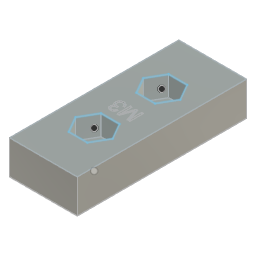
Joints v5 (Autodesk Fusion 360 design; units mm, degrees)
Autodesk Fusion 360 part; units mm, degrees
box "BoxPrimitive3" add length 5 width 10 height 25 placed x (0, 0, 1) y (1, 0, 0) z (0, 1, 0) at (0, 0, 0)
sketch "Sketch5" plane through (0, 0, 5) normal (0, 0, 1) x (-1, 0, 0)
  line L0 (0, -25) -> (0, 0)
  line L1 (0, 0) -> (-10, 0)
  line L2 (-10, 0) -> (-10, -25)
  line L3 (-10, -25) -> (0, -25)
  line L4 (-7.75, -7.5) -> (-6.375, -9.8816)
  line L5 (-6.375, -9.8816) -> (-3.625, -9.8816)
  line L6 (-3.625, -9.8816) -> (-2.25, -7.5)
  line L7 (-2.25, -7.5) -> (-3.625, -5.1184)
  line L8 (-3.625, -5.1184) -> (-6.375, -5.1184)
  line L9 (-6.375, -5.1184) -> (-7.75, -7.5)
  line L10 (-7.75, -17.5) -> (-6.375, -19.8816)
  line L11 (-6.375, -19.8816) -> (-3.625, -19.8816)
  line L12 (-3.625, -19.8816) -> (-2.25, -17.5)
  line L13 (-2.25, -17.5) -> (-3.625, -15.1184)
  line L14 (-3.625, -15.1184) -> (-6.375, -15.1184)
  line L15 (-6.375, -15.1184) -> (-7.75, -17.5)
  point P0 (-5, -17.5)
  point P1 (-5, -7.5)
  point P2 (-5, -17.5)
  point P3 (-5, -7.5)
  point P4 (-5, -17.5)
  point P5 (-5, -7.5)
  dimension "d23" = 2.75
  dimension "d24" = 2.75
  constraint coincident P4 P2
  constraint coincident P5 P3
  measures "d23" distance of L4.start P5
  measures "d24" distance of L10.start P4
extrude "Extrude3" cut sketch "Sketch5" against normal blind 3 contours L4 L5 L6 L7 L8 L9 | L10 L11 L12 L13 L14 L15
sketch "Sketch7" plane through (0, 0, 5) normal (0, 0, 1) x (-1, 0, 0)
  line L0 (-6.375, -19.8816) -> (-7.75, -17.5)
  line L1 (-7.75, -17.5) -> (-6.375, -15.1184)
  line L2 (-6.375, -15.1184) -> (-3.625, -15.1184)
  line L3 (-3.625, -15.1184) -> (-2.25, -17.5)
  line L4 (-2.25, -17.5) -> (-3.625, -19.8816)
  line L5 (-3.625, -19.8816) -> (-6.375, -19.8816)
  line L6 (-6.375, -9.8816) -> (-7.75, -7.5)
  line L7 (-7.75, -7.5) -> (-6.375, -5.1184)
  line L8 (-6.375, -5.1184) -> (-3.625, -5.1184)
  line L9 (-3.625, -5.1184) -> (-2.25, -7.5)
  line L10 (-2.25, -7.5) -> (-3.625, -9.8816)
  line L11 (-3.625, -9.8816) -> (-6.375, -9.8816)
  line L12 (0, -25) -> (0, 0)
  line L13 (0, 0) -> (-10, 0)
  line L14 (-10, 0) -> (-10, -25)
  line L15 (-10, -25) -> (0, -25)
  circle A0 centre (-5, -7.5) radius 1.5
  dimension "d27" = 3
  measures "d27" diameter of A0
extrude "Extrude4" cut sketch "Sketch7" against normal blind 5 contours A0
cylinder "CylinderPrimitive1" cut diameter 3 height -5 placed x (1, 0, 0) y (0, 1, 0) z (0, 0, 1) at (5, 17.5, 5)
sketch "Sketch9" plane through (0, 0, 5) normal (0, 0, 1) x (1, 0, 0)
  line L0 (7.5, 13, 1) -> (2.5, 13, 1) construction
  line L1 (2.5, 13, 1) -> (2.5, 11, 1) construction
  line L2 (2.5, 11, 1) -> (7.5, 11, 1) construction
  line L3 (7.5, 11, 1) -> (7.5, 13, 1) construction
  dimension "d32" = 2
  text T0 "M3" font "Arial" height 2 align centre top in box 5 x 2 at (7.5, 13) x (-1, 0) y (0, -1) spacing 1 kerned
emboss "Emboss1" depth -0.25 profiles "Sketch9" section 1 text T0 onto face at (5.4583, 23.2939, 5)
sketch "Sketch6" plane through (0, 0, 0) normal (1, 0, 0) x (0, 1, 0)
  point P0 (12, 0)
